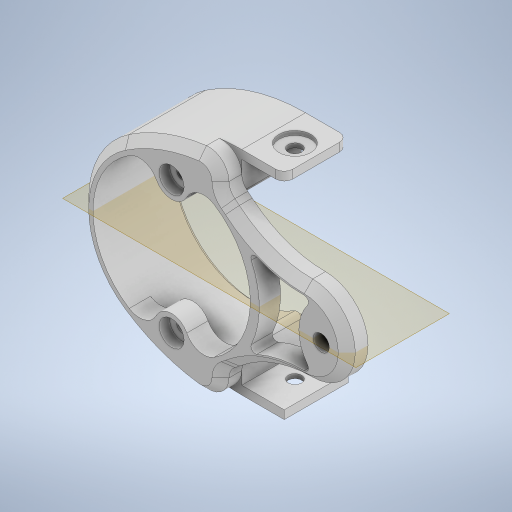
# Autodesk Inventor part: Wheel_Bracket_2
Saved by Autodesk Inventor 2024 (Build 280153000, 153)
## iProperties
Created: 2024-04-12
Part Number: Wheel_Bracket_2
Material: Generic
Document SubType Name: Modeling
Designer: CJ110
Density: 1 g/cm^3
Appearance: Default
Author: CJ110
Autodesk Inventor part; units mm, degrees
ref_plane "YZ Plane" through (0, 0, 0) normal (1, 0, 0) x (0, 1, 0)
ref_plane "XZ Plane" through (0, 0, 0) normal (0, 1, 0) x (-1, 0, 0)
ref_plane "XY Plane" through (0, 0, 0) normal (0, 0, 1) x (1, 0, 0)
sketch "Sketch1" plane through (0, 0, 0) normal (0, 0, 1) x (1, 0, 0)
  circle A0 centre (0, 0) radius 18.5
  line L0 (-21.5, 25) -> (-11.5, 25)
  line L1 (-11.5, 25) -> (-11.5, 23)
  line L2 (-11.5, 23) -> (-21.5, 23)
  line L3 (-21.5, 23) -> (-21.5, 25)
  line L4 (-21.5, -23) -> (-11.5, -23)
  line L5 (-11.5, -23) -> (-11.5, -25)
  line L6 (-11.5, -25) -> (-21.5, -25)
  line L7 (-21.5, -25) -> (-21.5, -23)
  circle A1 centre (0, 0) radius 21.5
  arc A2 (11.9775, 17.8547) -> (-11.5, 25) centre (-11.5, -17.1429) ccw
  arc A3 (-11.5, -25) -> (11.9775, -17.8547) centre (-11.5, 17.1429) ccw
  line L8 (0, 0) -> (-21.5, 0) construction
  line L9 (-11.5, 23) -> (-11.5, -23)
  point P0 (-11.5, 0)
  point P1 (-21.5, 24)
  point P2 (-11.5, 14.4914)
  point P3 (-11.5, -14.4914)
  dimension "d0" = 37
  dimension "d2" = 50
  dimension "d3" = 2
  dimension "d4" = 43
  dimension "d5" = 10
  constraints: 20 end point, 7 point on circle, 4 centre point, 4 parallel, 4 tangent, 3 horizontal, 3 perpendicular, 2 coincident, 2 equal length, 2 midpoint, 1 point on line, 1 vertical alignment
  measures "d0" diameter of A0
  measures "d2" distance between parallel lines of L6 L0
  measures "d3" distance between parallel lines of L4 L6
  measures "d4" diameter of A1
  measures "d5" distance of L1.end L2.end
extrude "Extrusion1" add sketch "Sketch1" along normal blind 15 contours A0 L9 A1 | L9 L1 A2 A1 | A1 A3 L5 L9 | L2 L3 L0 L1 | L5 L6 L7 L4 picked at (20.286, -1.7382)
ref_plane "Work Plane1" through (-21.5, 0, 0) normal (0, 1, 0) x (1, 0, 0)
sketch "Sketch2" plane through (0, 0, 0) normal (0, 0, -1) x (-1, 0, 0)
  line L0 (0, 18.5) -> (0, -18.5) construction
  line L1 (21.5, 25) -> (21.5, 23) projected
  line L2 (11.5, 25) -> (21.5, 25) projected
  arc A0 (11.5, 25) -> (-11.9775, 17.8547) centre (11.5, -17.1429) ccw projected
  arc A1 (-11.9775, 17.8547) -> (-11.9775, -17.8547) centre (0, 0) ccw projected
  arc A2 (-11.9775, -17.8547) -> (11.5, -25) centre (11.5, 17.1429) ccw projected
  line L3 (21.5, -25) -> (11.5, -25) projected
  line L4 (21.5, -23) -> (21.5, -25) projected
  line L5 (11.5, -23) -> (21.5, -23) projected
  line L6 (11.5, -14.4914) -> (11.5, -23) projected
  arc A3 (11.5, 14.4914) -> (11.5, -14.4914) centre (0, 0) ccw projected
  line L7 (11.5, 23) -> (11.5, 14.4914) projected
  line L8 (21.5, 23) -> (11.5, 23) projected
  circle A4 centre (0, -15.6) radius 1.27
  circle A5 centre (0, -15.6) radius 4
  arc A6 (3.5821, -13.82) -> (9.9615, -15.589) centre (7.5661, -11.8403) ccw
  arc A7 (11.5, 14.4914) -> (11.5, -14.4914) centre (0, 0) ccw projected
  circle A8 centre (10.5, -16.4317) radius 1
  arc A9 (-9.9615, -15.589) -> (-3.5821, -13.82) centre (-7.5661, -11.8403) ccw
  circle A10 centre (0, 0) radius 21.5
  circle A11 centre (0, 0) radius 18.5
  line L9 (19.0329, -10) -> (41.2, -10)
  line L10 (41.2, -10) -> (41.2, 10)
  line L11 (41.2, 10) -> (19.0329, 10)
  circle A12 centre (35.2, 0) radius 1.905
  arc A13 (31.2, -10) -> (41.2, 0) centre (31.2, 0) ccw
  arc A14 (41.2, 0) -> (31.2, 10) centre (31.2, 0) ccw
  arc A15 (13.9536, 16.3568) -> (31.2, 10) centre (31.2, 36.5735) ccw
  arc A16 (11.5, -20) -> (14.5, -23) centre (14.5, -20) ccw
  line L12 (11.5, -23) -> (21.5, -23) projected
  arc A17 (12.9, -17.2) -> (11.5, -20) centre (15, -20) ccw
  line L13 (11.5, -14.4914) -> (11.5, -23) projected
  arc A18 (31.2, -10) -> (13.9536, -16.3568) centre (31.2, -36.5735) ccw
  arc A19 (14.5, 23) -> (11.5, 20) centre (14.5, 20) ccw
  arc A20 (11.5, 20) -> (12.9, 17.2) centre (15, 20) ccw
  line L14 (11.5, 23) -> (11.5, 14.4914) projected
  line L15 (11.5, 23) -> (11.5, 25)
  line L16 (11.5, -23) -> (11.5, -25)
  arc A21 (11.5, 20) -> (6.2057, 24.6661) centre (6.7966, 20) ccw
  arc A22 (11.5, 25) -> (-11.9775, 17.8547) centre (11.5, -17.1429) ccw projected
  arc A23 (6.2057, -24.6661) -> (11.5, -20) centre (6.7966, -20) ccw
  arc A24 (-11.9775, -17.8547) -> (11.5, -25) centre (11.5, 17.1429) ccw projected
  point P0 (-11.9775, 17.8547)
  point P1 (-11.9775, -17.8547)
  point P2 (-9.9615, -15.589)
  point P3 (11.5, 14.4914)
  point P4 (-11.9775, 17.8547)
  point P5 (11.5, 18.1659)
  point P6 (11.5, -18.1659)
  point P7 (-11.9775, -17.8547)
  point P8 (11.5, -16.4317)
  dimension "d11" = 2
  dimension "d8" = 2.54
  dimension "d9" = 15.6
  dimension "d10" = 8
  dimension "d12" = 35.2
  dimension "d13" = 3.81
  dimension "d14" = 20
  dimension "d15" = 6
  dimension "d23" = 3
  dimension "d24" = 3
  constraints: 38 point on circle, 25 tangent, 17 centre point, 12 end point, 7 point on line, 3 coincident, 3 equal radius, 3 midpoint, 3 vertical, 2 horizontal alignment, 2 perpendicular, 1 collinear, 1 horizontal, 4 other
  measures "d8" diameter of A4
  measures "d9" distance of point (0, 0) A4.centre
  measures "d10" diameter of A5
  measures "d12" distance of point (0, 0) A12.centre
  measures "d13" diameter of A12
  measures "d14" distance of L9.end L10.end
  measures "d15" distance of A12.centre A13.end
  measures "d23" distance from line of L5 A16.start
  measures "d24" distance from line of L8 A19.end
extrude "Extrusion2" add sketch "Sketch2" along normal blind 5 contours A21 L7 A10 A0 | A20 A10 L7 | A10 L7 A3 A5 A8 L6 A1 | A10 L6 A11 L7 | A10 L6 A23 A2 | A15 L11 A10 | A10 A17 L6 | L11 A14 A13 L9 A10 | A8 A3 L6 | A8 | A3 A5 | A10 L9 A18 picked at (0.1604, -18.8389)
extrude "Extrusion3" add sketch "Sketch2" along normal blind 5 contours A9 A5 A3 | A5 A3 | A3 A5 A6 picked at (-1.6472, -17.724)
sketch "Sketch3" plane through (0, 0, -5) normal (0, 0, -1) x (-1, 0, 0)
  circle A0 centre (0, -15.6) radius 1.27 projected
  arc A1 (9.9615, -15.589) -> (-9.9615, -15.589) centre (0, 0) ccw projected
  arc A2 (3.5821, -13.82) -> (9.9615, -15.589) centre (7.5661, -11.8403) ccw projected
  arc A3 (3.5821, -13.82) -> (-3.5821, -13.82) centre (0, -15.6) ccw projected
  arc A4 (-9.9615, -15.589) -> (-3.5821, -13.82) centre (-7.5661, -11.8403) ccw projected
  circle A5 centre (0, -15.6) radius 2.95
  arc A6 (6.2057, 24.6661) -> (-11.9775, 17.8547) centre (11.5, -17.1429) ccw projected
  arc A7 (-11.9775, 17.8547) -> (-11.9775, -17.8547) centre (0, 0) ccw projected
  arc A8 (-11.9775, -17.8547) -> (6.2057, -24.6661) centre (11.5, 17.1429) ccw projected
  arc A9 (13.9536, 16.3568) -> (12.9, 17.2) centre (0, 0) ccw projected
  arc A10 (12.9, -17.2) -> (11.5, -20) centre (15, -20) ccw projected
  arc A11 (12.9, -17.2) -> (13.9536, -16.3568) centre (0, 0) ccw projected
  arc A12 (31.2, -10) -> (13.9536, -16.3568) centre (31.2, -36.5735) ccw projected
  arc A13 (13.9536, 16.3568) -> (31.2, 10) centre (31.2, 36.5735) ccw projected
  arc A14 (31.2, -10) -> (31.2, 10) centre (31.2, 0) ccw projected
  arc A15 (11.5, 20) -> (12.9, 17.2) centre (15, 20) ccw projected
  arc A16 (11.5, 20) -> (6.2057, 24.6661) centre (6.7966, 20) ccw projected
  arc A17 (6.2057, -24.6661) -> (11.5, -20) centre (6.7966, -20) ccw projected
  dimension "d20" = 5.9
  constraints: 1 centre point, 1 coincident
  measures "d20" diameter of A5
extrude "Extrusion4" cut sketch "Sketch3" against normal blind 2.5 contours A5
mirror "Mirror2" about plane through (-21.5, 0, 0) normal (0, 1, 0) of "Extrusion4", "Extrusion3"
sketch "Sketch4" plane through (0, 0, -5) normal (0, 0, -1) x (-1, 0, 0)
  circle A0 centre (19.6584, 9) radius 1
  circle A1 centre (19.6584, -9) radius 1
  arc A2 (18.7491, -8.5837) -> (18.7491, 8.5837) centre (0, 0) ccw
  circle A3 centre (31.2, 6.6816) radius 1
  circle A4 centre (31.2, -6.6816) radius 1
  arc A5 (31.9944, 6.0742) -> (31.9944, -6.0742) centre (39.9382, 0) ccw
  arc A6 (20.0601, 9.9158) -> (31.1831, 7.6814) centre (30.7344, 34.2511) ccw
  arc A7 (31.1831, -7.6814) -> (20.0601, -9.9158) centre (30.7344, -34.2511) ccw
  line L0 (-34.04, 0) -> (53.74, 0) projected
  circle A8 centre (35.2, 0) radius 1.905 projected
  arc A9 (9.9615, -15.589) -> (9.9615, 15.589) centre (0, 0) ccw projected
  circle A10 centre (0, 15.6) radius 2.95 projected
  circle A11 centre (0, -15.6) radius 2.95 projected
  arc A12 (-11.9775, 17.8547) -> (-11.9775, -17.8547) centre (0, 0) ccw projected
  arc A13 (-11.9775, -17.8547) -> (6.2057, -24.6661) centre (11.5, 17.1429) ccw projected
  arc A14 (12.9, -17.2) -> (11.5, -20) centre (15, -20) ccw projected
  arc A15 (12.9, -17.2) -> (13.9536, -16.3568) centre (0, 0) ccw projected
  arc A16 (31.2, -10) -> (13.9536, -16.3568) centre (31.2, -36.5735) ccw projected
  arc A17 (31.2, -10) -> (31.2, 10) centre (31.2, 0) ccw projected
  arc A18 (13.9536, 16.3568) -> (31.2, 10) centre (31.2, 36.5735) ccw projected
  arc A19 (13.9536, 16.3568) -> (12.9, 17.2) centre (0, 0) ccw projected
  arc A20 (11.5, 20) -> (12.9, 17.2) centre (15, 20) ccw projected
  arc A21 (6.2057, 24.6661) -> (-11.9775, 17.8547) centre (11.5, -17.1429) ccw projected
  arc A22 (-9.9615, 15.589) -> (-9.9615, -15.589) centre (0, 0) ccw projected
  arc A23 (-3.5821, 13.82) -> (-9.9615, 15.589) centre (-7.5661, 11.8403) ccw projected
  arc A24 (-3.5821, 13.82) -> (3.5821, 13.82) centre (0, 15.6) ccw projected
  arc A25 (9.9615, 15.589) -> (3.5821, 13.82) centre (7.5661, 11.8403) ccw projected
  arc A26 (9.9615, -15.589) -> (9.9615, 15.589) centre (0, 0) ccw projected
  arc A27 (3.5821, -13.82) -> (9.9615, -15.589) centre (7.5661, -11.8403) ccw projected
  arc A28 (3.5821, -13.82) -> (-3.5821, -13.82) centre (0, -15.6) ccw projected
  arc A29 (-9.9615, -15.589) -> (-3.5821, -13.82) centre (-7.5661, -11.8403) ccw projected
  circle A30 centre (35.2, 0) radius 1.905 projected
  arc A31 (11.5, 20) -> (6.2057, 24.6661) centre (6.7966, 20) ccw projected
  arc A32 (6.2057, -24.6661) -> (11.5, -20) centre (6.7966, -20) ccw projected
  arc A33 (13.9536, 16.3568) -> (31.2, 10) centre (31.2, 36.5735) ccw projected
  line L1 (17.3825, 6.3322) -> (21.9342, 11.6678) construction
  line L2 (0, 0) -> (13.9536, 16.3568) construction
  line L3 (20.0601, 9.9158) -> (20.9914, 12.0391) construction
  line L4 (31.1831, 7.6814) -> (31.2, 10) construction
  dimension "d25" = 2
  dimension "d26" = 4
  dimension "d28" = 10
  dimension "d30" = 18
  constraints: 19 point on circle, 8 centre point, 8 end point, 8 tangent, 5 equal radius, 2 point on line, 2 vertical alignment, 1 coincident, 1 concentric, 1 equal length, 1 line through centre, 1 midpoint, 1 parallel
  measures "d25" diameter of A3
  measures "d26" horizontal distance of A4.centre A8.centre
  measures "d28" radius of A5
  measures "d30" distance of A1.centre A0.centre
extrude "Extrusion5" cut sketch "Sketch4" against normal up to next contours A0 | A0 A6 A3 A5 L0 A2 | A3 | L0 A5 A4 A7 A1 A2 | A1 | A4
extrude "Extrusion6" cut sketch "Sketch2" against normal up to next contours A8 A3 L6
mirror "Mirror3" about plane through (-21.5, 0, 0) normal (0, 1, 0) of "Extrusion6"
sketch "Sketch5" plane through (-21.5, 25, 15) normal (0, 1, 0) x (1, 0, 0)
  circle A0 centre (5, 7.5) radius 1.59
  line L0 (10, 15) -> (0, 15) projected
  line L1 (0, 15) -> (0, 0) projected
  line L2 (10, 0) -> (0, 0) projected
  line L3 (10, 15) -> (10, 0) projected
  line L4 (0, 7.5) -> (10, 7.5) construction
  point P0 (21.5, 15)
  dimension "d36" = 3.18
  dimension "d37" = 5
  constraints: 3 midpoint, 2 end point, 1 centre point
  measures "d36" diameter of A0
  measures "d37" distance from line of L1 A0.centre
extrude "Extrusion7" cut sketch "Sketch5" against normal through all contours A0
sketch "Sketch6" plane through (-21.5, 25, 0) normal (0, 1, 0) x (1, 0, 0)
  circle A0 centre (5, -7.5) radius 1.59 projected
  line L0 (10, 0) -> (0, 0) projected
  line L1 (0, 0) -> (0, -15) projected
  line L2 (10, -15) -> (0, -15) projected
  line L3 (10, 0) -> (10, -15) projected
  circle A1 centre (5, -7.5) radius 3.75
  point P0 (21.5, 0)
  dimension "d40" = 7.5
  constraints: 1 centre point, 1 coincident
  measures "d40" diameter of A1
extrude "Extrusion8" cut sketch "Sketch6" against normal blind 1 contours A1
mirror "Mirror4" about plane through (-21.5, 0, 0) normal (0, 1, 0) of "Extrusion8"
chamfer "Chamfer1" distance 2 angle 45 12 edges at (3.2835, 22.3219, -5) (21.5, 0, -5) (3.2835, -22.3219, -5) (-9.9065, -23.5285, -5) (-11.8695, -18.4348, -5) (-13.4334, -16.7867, -5) (-22.0097, -11.6398, -5) (-41.2, 0, -5) (-22.0097, 11.6398, -5) (-13.4334, 16.7867, -5) (-11.8695, 18.4348, -5) (-9.9065, 23.5285, -5)
fillet "Fillet1" radius 2 2 edges at (-21.5, 24, 0) (-21.5, 24, 15)
chamfer "Chamfer2" distance 1 angle 45 5 edges at (18.5, 0, 15) (-10.9804, -15.5546, 15) (-11.5, -19.7158, 15) (-10.9804, 15.5546, 15) (-11.5, 19.7158, 15)
body "Solid1"
